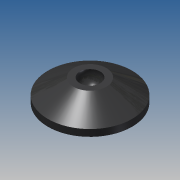
# Autodesk Inventor part: Plastikfuß_40mm
Saved by Autodesk Inventor 2015 (Build 190159000, 159)
## iProperties
Created: 2015-01-09
Part Number: Plastikfuß_40mm
Material: ABS-Kunststoff
Document SubType Name: Modeling
Designer: Marc
Mass: 8.82723 g
Surface Area: 32.0917 cm^2
Volume: 8.32758 cm^3
Density: 1.06 g/cm^3
Appearance: Dunkelgrau
Author: Marc
Autodesk Inventor part; units mm, degrees
ref_plane "YZ Plane" through (0, 0, 0) normal (1, 0, 0) x (0, 1, 0)
ref_plane "XZ Plane" through (0, 0, 0) normal (0, 1, 0) x (-1, 0, 0)
sketch "Skizze1" plane through (0, 0, 0) normal (0, 0, 1) x (1, 0, 0)
  line L0 (0, -28) -> (0, 28) projected
  line L1 (-28, 0) -> (28, 0) projected
  circle A0 centre (0, 0) radius 20
  dimension "d0" = 40
  constraints: 1 centre point, 1 coincident
  measures "d0" diameter of A0
extrude "Extrusion1" add sketch "Skizze1" along normal mid plane 10.4
ref_plane "Arbeitsebene1" through (0, 0, 4) normal (0, 0, 1) x (1, 0, 0)
sketch "Skizze3" plane through (0, 0, 4) normal (0, 0, 1) x (1, 0, 0)
  arc A0 (-5, 0) -> (5, 0) centre (0, 0) ccw
  line L0 (-28, 0) -> (28, 0) projected
  line L1 (-5, 0) -> (5, 0)
  dimension "d4" = 10
  constraints: 2 end point, 2 point on circle, 2 point on line, 1 centre point, 1 coincident, 1 collinear
  measures "d4" diameter of A0
revolve "Umdrehung1" cut sketch "Skizze3" angle 360 about axis through (-10, 0, 4) along (1, 0, 0)
sketch "Skizze4" plane through (0, 0, 0) normal (0, 1, 0) x (-1, 0, 0)
  line L0 (-20, -5.2) -> (20, -5.2) projected
  line L1 (20, 5.2) -> (-20, 5.2) projected
  line L2 (-20, -5.2) -> (-20, 5.2) projected
  line L3 (28, 0) -> (-28, 0) projected
  line L4 (0, -7.28) -> (0, 7.28) projected
  line L5 (20, 5.2) -> (-20, 5.2) projected
  line L6 (-7.8, 5.2) -> (-20, -1.9841)
  line L7 (-20, -1.9841) -> (-20, 5.2)
  line L8 (-20, 5.2) -> (-7.8, 5.2)
  point P0 (0, 0)
  constraints: 6 end point, 2 point on line, 1 perpendicular
revolve "Umdrehung2" cut sketch "Skizze4" angle 360 about axis through (0, 0, -10) along (0, 0, 1) contours L2 L3 L6 | L2 L1 L6 L3
